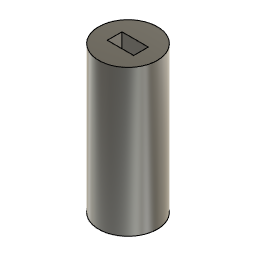
digital fabrication v1 (Autodesk Fusion 360 design; units mm, degrees)
Autodesk Fusion 360 part; units mm, degrees
sketch "Sketch1" plane through (0, 0, 0) normal (0, 0, 1) x (1, 0, 0) in component "ADAPTERI2"
  circle A0 centre (0, 0) radius 15
  dimension "d3" = 30
  constraint coincident A0.centre origin
  measures "d3" diameter of A0
extrude "Extrude1" add sketch "Sketch1" along normal blind 50 in component "ADAPTERI2"
sketch "Sketch2" plane through (-0.004, -0.0691, 50) normal (0, 0, 1) x (-1, 0, 0) in component "ADAPTERI2"
  circle A0 centre (-0.004, -0.0691) radius 15
  line L0 (-4.5, 2.5) -> (4.5, 2.5)
  line L1 (4.5, 2.5) -> (4.5, -2.5)
  line L2 (4.5, -2.5) -> (-4.5, -2.5)
  line L3 (-4.5, -2.5) -> (-4.5, 2.5)
  line L4 (-4.5, 2.5) -> (4.5, -2.5) construction
  line L5 (4.5, 2.5) -> (-4.5, -2.5) construction
  dimension "d6" = 9
  dimension "d7" = 5
  constraint horizontal L0
  constraint perpendicular L0 L1
  constraint parallel L0 L2
  constraint parallel L1 L3
  constraint coincident L4 origin
  constraint coincident L5 origin
  measures "d6" distance of L1.end L2.end
  measures "d7" distance of L0.end L1.end
extrude "Extrude2" cut sketch "Sketch2" against normal blind 10 contours L0 L1 L2 L3 in component "ADAPTERI2"
sketch "Sketch3" plane through (-0.2192, -4.1274, 0) normal (0, 0, -1) x (1, 0, 0) in component "ADAPTERI2"
  circle A0 centre (0.2192, -4.1274) radius 15
  line L0 (0.3727, -11.0539) -> (6.2945, -7.4577)
  line L1 (6.2945, -7.4577) -> (6.1409, -0.5312)
  line L2 (6.1409, -0.5312) -> (0.0656, 2.7991)
  line L3 (0.0656, 2.7991) -> (-5.8561, -0.7971)
  line L4 (-5.8561, -0.7971) -> (-5.7026, -7.7236)
  line L5 (-5.7026, -7.7236) -> (0.3727, -11.0539)
  point P0 (0.2192, -4.1274)
  dimension "d10" = 6
  constraint coincident P0 A0.centre
  measures "d10" distance of P0 L5
extrude "Extrude3" cut sketch "Sketch3" against normal blind 20 contours L0 L1 L2 L3 L4 L5 in component "ADAPTERI2"
move_face "OffsetFaces1" offset -5 1 faces at (14.9255, -1.4935, 16.6667) in component "ADAPTERI2"
component "ADAPTERI2" placed x (1, 0, 0) y (0, 1, 0) z (0, 0, 1) at (0, 0, 0)
